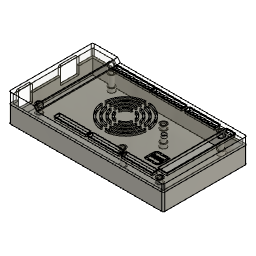
CaseArduino_MicaelMarques_2021.1 (Autodesk Fusion 360 design; units mm, degrees)
Autodesk Fusion 360 part; units mm, degrees
note: some values were not read from the file. Set by a fixed rule: which face or edge a step refers to.
sketch "Sketch1" plane through (0, 0, 0) normal (0, 0, 1) x (1, 0, 0)
  line L0 (-51.8, 28.67) -> (51.8, 28.67)
  line L1 (52.8, 27.67) -> (52.8, -27.67)
  line L2 (51.8, -28.67) -> (-51.8, -28.67)
  line L3 (-52.8, -27.67) -> (-52.8, 27.67)
  line L4 (-52.8, 28.67) -> (52.8, -28.67) construction
  line L5 (52.8, 28.67) -> (-52.8, -28.67) construction
  line L6 (-1.55, -22.32) -> (19.37, -22.32)
  line L7 (19.57, -22.52) -> (19.57, -25.53)
  line L8 (19.37, -25.73) -> (-1.55, -25.73)
  line L9 (-1.75, -25.53) -> (-1.75, -22.52)
  line L10 (21.31, -22.32) -> (42.23, -22.32)
  line L11 (42.43, -22.52) -> (42.43, -25.53)
  line L12 (42.23, -25.73) -> (21.31, -25.73)
  line L13 (21.11, -25.53) -> (21.11, -22.52)
  line L14 (-33.25, 25.94) -> (-7.85, 25.94)
  line L15 (-7.65, 25.74) -> (-7.65, 22.73)
  line L16 (-7.85, 22.53) -> (-33.25, 22.53)
  line L17 (-33.45, 22.73) -> (-33.45, 25.74)
  line L18 (-6.33, 25.94) -> (13.99, 25.94)
  line L19 (14.19, 25.74) -> (14.19, 22.73)
  line L20 (13.99, 22.53) -> (-6.33, 22.53)
  line L21 (-6.53, 22.73) -> (-6.53, 25.74)
  line L22 (16.53, 25.94) -> (36.85, 25.94)
  line L23 (37.05, 25.74) -> (37.05, 22.73)
  line L24 (36.85, 22.53) -> (16.53, 22.53)
  line L25 (16.33, 22.73) -> (16.33, 25.74)
  line L26 (41.69, 25.94) -> (47.24, 25.94)
  line L27 (47.44, 25.74) -> (47.44, -20.58)
  line L28 (47.24, -20.78) -> (41.69, -20.78)
  line L29 (41.49, -20.58) -> (41.49, 25.74)
  line L30 (-24.41, -22.32) -> (-3.49, -22.32)
  line L31 (-3.29, -22.52) -> (-3.29, -25.53)
  line L32 (-3.49, -25.73) -> (-24.41, -25.73)
  line L33 (-24.61, -25.53) -> (-24.61, -22.52)
  circle A0 centre (-36.81, -24.02) radius 2.2
  circle A1 centre (15.26, 9) radius 2.2
  circle A2 centre (15.26, -18.94) radius 2.2
  circle A3 centre (39.39, 24.24) radius 2.2
  circle A4 centre (45.74, -24.02) radius 2.2
  circle A5 centre (-36.81, -24.02) radius 1.5
  circle A6 centre (15.26, 9) radius 1.5
  circle A7 centre (15.26, -18.94) radius 1.5
  circle A8 centre (39.39, 24.24) radius 1.5
  circle A9 centre (45.74, -24.02) radius 1.5
  circle A10 centre (-35.54, 24.24) radius 2.2
  circle A11 centre (-35.54, 24.24) radius 1.5
  arc A12 (-33.25, 25.94) -> (-33.45, 25.74) centre (-33.25, 25.74) ccw
  arc A13 (-33.45, 22.73) -> (-33.25, 22.53) centre (-33.25, 22.73) ccw
  arc A14 (-7.85, 22.53) -> (-7.65, 22.73) centre (-7.85, 22.73) ccw
  arc A15 (-7.65, 25.74) -> (-7.85, 25.94) centre (-7.85, 25.74) ccw
  arc A16 (-6.33, 25.94) -> (-6.53, 25.74) centre (-6.33, 25.74) ccw
  arc A17 (-6.53, 22.73) -> (-6.33, 22.53) centre (-6.33, 22.73) ccw
  arc A18 (13.99, 22.53) -> (14.19, 22.73) centre (13.99, 22.73) ccw
  arc A19 (14.19, 25.74) -> (13.99, 25.94) centre (13.99, 25.74) ccw
  arc A20 (16.53, 25.94) -> (16.33, 25.74) centre (16.53, 25.74) ccw
  arc A21 (16.33, 22.73) -> (16.53, 22.53) centre (16.53, 22.73) ccw
  arc A22 (36.85, 22.53) -> (37.05, 22.73) centre (36.85, 22.73) ccw
  arc A23 (37.05, 25.74) -> (36.85, 25.94) centre (36.85, 25.74) ccw
  arc A24 (41.69, 25.94) -> (41.49, 25.74) centre (41.69, 25.74) ccw
  arc A25 (47.44, 25.74) -> (47.24, 25.94) centre (47.24, 25.74) ccw
  arc A26 (41.49, -20.58) -> (41.69, -20.78) centre (41.69, -20.58) ccw
  arc A27 (47.24, -20.78) -> (47.44, -20.58) centre (47.24, -20.58) ccw
  arc A28 (21.31, -22.32) -> (21.11, -22.52) centre (21.31, -22.52) ccw
  arc A29 (21.11, -25.53) -> (21.31, -25.73) centre (21.31, -25.53) ccw
  arc A30 (42.23, -25.73) -> (42.43, -25.53) centre (42.23, -25.53) ccw
  arc A31 (42.43, -22.52) -> (42.23, -22.32) centre (42.23, -22.52) ccw
  arc A32 (-1.55, -22.32) -> (-1.75, -22.52) centre (-1.55, -22.52) ccw
  arc A33 (-1.75, -25.53) -> (-1.55, -25.73) centre (-1.55, -25.53) ccw
  arc A34 (19.37, -25.73) -> (19.57, -25.53) centre (19.37, -25.53) ccw
  arc A35 (19.57, -22.52) -> (19.37, -22.32) centre (19.37, -22.52) ccw
  arc A36 (-24.41, -22.32) -> (-24.61, -22.52) centre (-24.41, -22.52) ccw
  arc A37 (-24.61, -25.53) -> (-24.41, -25.73) centre (-24.41, -25.53) ccw
  arc A38 (-3.49, -25.73) -> (-3.29, -25.53) centre (-3.49, -25.53) ccw
  arc A39 (-3.29, -22.52) -> (-3.49, -22.32) centre (-3.49, -22.52) ccw
  arc A40 (-33.75, 22.73) -> (-33.25, 22.23) centre (-33.25, 22.73) ccw
  line L34 (-7.85, 22.23) -> (-33.25, 22.23)
  arc A41 (-7.85, 22.23) -> (-7.35, 22.73) centre (-7.85, 22.73) ccw
  line L35 (-7.35, 25.74) -> (-7.35, 22.73)
  arc A42 (-7.35, 25.74) -> (-7.85, 26.24) centre (-7.85, 25.74) ccw
  line L36 (-33.25, 26.24) -> (-7.85, 26.24)
  arc A43 (-33.25, 26.24) -> (-33.75, 25.74) centre (-33.25, 25.74) ccw
  line L37 (-33.75, 22.73) -> (-33.75, 25.74)
  arc A44 (-6.83, 22.73) -> (-6.33, 22.23) centre (-6.33, 22.73) ccw
  line L38 (13.99, 22.23) -> (-6.33, 22.23)
  arc A45 (13.99, 22.23) -> (14.49, 22.73) centre (13.99, 22.73) ccw
  line L39 (14.49, 25.74) -> (14.49, 22.73)
  arc A46 (14.49, 25.74) -> (13.99, 26.24) centre (13.99, 25.74) ccw
  line L40 (-6.33, 26.24) -> (13.99, 26.24)
  arc A47 (-6.33, 26.24) -> (-6.83, 25.74) centre (-6.33, 25.74) ccw
  line L41 (-6.83, 22.73) -> (-6.83, 25.74)
  arc A48 (37.35, 25.74) -> (36.85, 26.24) centre (36.85, 25.74) ccw
  line L42 (16.53, 26.24) -> (36.85, 26.24)
  arc A49 (16.53, 26.24) -> (16.03, 25.74) centre (16.53, 25.74) ccw
  line L43 (16.03, 22.73) -> (16.03, 25.74)
  arc A50 (16.03, 22.73) -> (16.53, 22.23) centre (16.53, 22.73) ccw
  line L44 (36.85, 22.23) -> (16.53, 22.23)
  arc A51 (36.85, 22.23) -> (37.35, 22.73) centre (36.85, 22.73) ccw
  line L45 (37.35, 25.74) -> (37.35, 22.73)
  arc A52 (41.69, 26.24) -> (41.19, 25.74) centre (41.69, 25.74) ccw
  line L46 (41.19, -20.58) -> (41.19, 25.74)
  arc A53 (41.19, -20.58) -> (41.69, -21.08) centre (41.69, -20.58) ccw
  line L47 (47.24, -21.08) -> (41.69, -21.08)
  arc A54 (47.24, -21.08) -> (47.74, -20.58) centre (47.24, -20.58) ccw
  line L48 (47.74, 25.74) -> (47.74, -20.58)
  arc A55 (47.74, 25.74) -> (47.24, 26.24) centre (47.24, 25.74) ccw
  line L49 (41.69, 26.24) -> (47.24, 26.24)
  arc A56 (42.73, -22.52) -> (42.23, -22.02) centre (42.23, -22.52) ccw
  line L50 (21.31, -22.02) -> (42.23, -22.02)
  arc A57 (21.31, -22.02) -> (20.81, -22.52) centre (21.31, -22.52) ccw
  line L51 (20.81, -25.53) -> (20.81, -22.52)
  arc A58 (20.81, -25.53) -> (21.31, -26.03) centre (21.31, -25.53) ccw
  line L52 (42.23, -26.03) -> (21.31, -26.03)
  arc A59 (42.23, -26.03) -> (42.73, -25.53) centre (42.23, -25.53) ccw
  line L53 (42.73, -22.52) -> (42.73, -25.53)
  arc A60 (19.87, -22.52) -> (19.37, -22.02) centre (19.37, -22.52) ccw
  line L54 (-1.55, -22.02) -> (19.37, -22.02)
  arc A61 (-1.55, -22.02) -> (-2.05, -22.52) centre (-1.55, -22.52) ccw
  line L55 (-2.05, -25.53) -> (-2.05, -22.52)
  arc A62 (-2.05, -25.53) -> (-1.55, -26.03) centre (-1.55, -25.53) ccw
  line L56 (19.37, -26.03) -> (-1.55, -26.03)
  arc A63 (19.37, -26.03) -> (19.87, -25.53) centre (19.37, -25.53) ccw
  line L57 (19.87, -22.52) -> (19.87, -25.53)
  arc A64 (-2.99, -22.52) -> (-3.49, -22.02) centre (-3.49, -22.52) ccw
  line L58 (-24.41, -22.02) -> (-3.49, -22.02)
  arc A65 (-24.41, -22.02) -> (-24.91, -22.52) centre (-24.41, -22.52) ccw
  line L59 (-24.91, -25.53) -> (-24.91, -22.52)
  arc A66 (-24.91, -25.53) -> (-24.41, -26.03) centre (-24.41, -25.53) ccw
  line L60 (-3.49, -26.03) -> (-24.41, -26.03)
  arc A67 (-3.49, -26.03) -> (-2.99, -25.53) centre (-3.49, -25.53) ccw
  line L61 (-2.99, -22.52) -> (-2.99, -25.53)
  arc A68 (-51.8, 28.67) -> (-52.8, 27.67) centre (-51.8, 27.67) ccw
  arc A69 (-52.8, -27.67) -> (-51.8, -28.67) centre (-51.8, -27.67) ccw
  arc A70 (51.8, -28.67) -> (52.8, -27.67) centre (51.8, -27.67) ccw
  line L62 (51.3, -27.17) -> (-51.3, -27.17) construction
  line L63 (-51.3, -27.17) -> (-51.3, 27.17) construction
  line L64 (-51.3, 27.17) -> (51.3, 27.17) construction
  line L65 (51.3, 27.17) -> (51.3, -27.17) construction
  arc A71 (52.8, 27.67) -> (51.8, 28.67) centre (51.8, 27.67) ccw
  dimension "d1" = 105.6
  dimension "d2" = 57.34
  dimension "d3" = 2.94
  dimension "d6" = 3.41
  dimension "d9" = 10.37
  dimension "d10" = 21.32
  dimension "d11" = 1.54
  dimension "d12" = 21.32
  dimension "d15" = 1.54
  dimension "d16" = 21.32
  dimension "d17" = 5.36
  dimension "d18" = 5.95
  dimension "d19" = 7.89
  dimension "d20" = 46.72
  dimension "d21" = 4.44
  dimension "d22" = 20.72
  dimension "d23" = 2.14
  dimension "d24" = 20.72
  dimension "d25" = 1.12
  dimension "d26" = 25.8
  dimension "d27" = 3.41
  dimension "d28" = 2.73
  dimension "d30" = 4.4
  dimension "d31" = 4.4
  dimension "d32" = 4.4
  dimension "d33" = 4.4
  dimension "d34" = 4.4
  dimension "d36" = 3
  dimension "d37" = 3
  dimension "d38" = 3
  dimension "d39" = 3
  dimension "d40" = 3
  dimension "d41" = 13.41
  dimension "d42" = 4.43
  dimension "d43" = 7.06
  dimension "d44" = 4.65
  dimension "d45" = 9.73
  dimension "d46" = 37.54
  dimension "d47" = 37.54
  dimension "d48" = 19.67
  dimension "d49" = 4.65
  dimension "d50" = 15.99
  dimension "d51" = 12.2
  dimension "d53" = 4.4
  dimension "d54" = 3
  dimension "d55" = 4.43
  dimension "d56" = 17.26
  dimension "d57" = 1.5
  dimension "d131" = 0.2
  dimension "d132" = 0.2
  dimension "d133" = 0.2
  dimension "d134" = 0.2
  dimension "d135" = 0.2
  dimension "d136" = 0.2
  dimension "d137" = 0.2
  dimension "d138" = -0.3
  dimension "d139" = -0.3
  dimension "d140" = -0.3
  dimension "d141" = -0.3
  dimension "d142" = -0.3
  dimension "d143" = -0.3
  dimension "d144" = -0.3
  dimension "d158" = 1
  constraint horizontal L0
  constraint perpendicular L0 L1
  constraint parallel L0 L2
  constraint parallel L1 L3
  constraint coincident L4 origin
  constraint coincident L5 origin
  constraint horizontal L6
  constraint vertical L7
  constraint horizontal L8
  constraint vertical L9
  constraint horizontal L10
  constraint vertical L11
  constraint horizontal L12
  constraint vertical L13
  constraint horizontal L14
  constraint vertical L15
  constraint horizontal L16
  constraint vertical L17
  constraint horizontal L18
  constraint vertical L19
  constraint horizontal L20
  constraint vertical L21
  constraint horizontal L22
  constraint vertical L23
  constraint horizontal L24
  constraint vertical L25
  constraint horizontal L26
  constraint vertical L27
  constraint horizontal L28
  constraint vertical L29
  constraint collinear L8 L12
  constraint collinear L6 L10
  constraint horizontal L30
  constraint vertical L31
  constraint horizontal L32
  constraint vertical L33
  constraint collinear L8 L32
  constraint collinear L6 L30
  constraint collinear L18 L22
  constraint collinear L14 L22
  constraint collinear L20 L24
  constraint collinear L16 L24
  constraint concentric A0 A5
  constraint concentric A1 A6
  constraint concentric A2 A7
  constraint concentric A3 A8
  constraint concentric A4 A9
  constraint concentric A10 A11
  constraint tangent L14 A12
  constraint tangent L17 A12
  constraint tangent L16 A13
  constraint tangent L17 A13
  constraint equal A12 A13
  constraint tangent L16 A14
  constraint tangent L15 A14
  constraint equal A12 A14
  constraint tangent L14 A15
  constraint tangent L15 A15
  constraint equal A12 A15
  constraint tangent L18 A16
  constraint tangent L21 A16
  constraint tangent L20 A17
  constraint tangent L21 A17
  constraint equal A16 A17
  constraint tangent L19 A18
  constraint tangent L20 A18
  constraint equal A16 A18
  constraint tangent L18 A19
  constraint tangent L19 A19
  constraint equal A16 A19
  constraint tangent L22 A20
  constraint tangent L25 A20
  constraint tangent L24 A21
  constraint tangent L25 A21
  constraint equal A20 A21
  constraint tangent L23 A22
  constraint tangent L24 A22
  constraint equal A20 A22
  constraint tangent L22 A23
  constraint tangent L23 A23
  constraint equal A20 A23
  constraint tangent L26 A24
  constraint tangent L29 A24
  constraint tangent L26 A25
  constraint tangent L27 A25
  constraint equal A24 A25
  constraint tangent L28 A26
  constraint tangent L29 A26
  constraint equal A24 A26
  constraint tangent L27 A27
  constraint tangent L28 A27
  constraint equal A24 A27
  constraint tangent L10 A28
  constraint tangent L13 A28
  constraint tangent L12 A29
  constraint tangent L13 A29
  constraint equal A28 A29
  constraint tangent L11 A30
  constraint tangent L12 A30
  constraint equal A28 A30
  constraint tangent L10 A31
  constraint tangent L11 A31
  constraint equal A28 A31
  constraint tangent L6 A32
  constraint tangent L9 A32
  constraint tangent L8 A33
  constraint tangent L9 A33
  constraint equal A32 A33
  constraint tangent L7 A34
  constraint tangent L8 A34
  constraint equal A32 A34
  constraint tangent L6 A35
  constraint tangent L7 A35
  constraint equal A32 A35
  constraint tangent L30 A36
  constraint tangent L33 A36
  constraint tangent L32 A37
  constraint tangent L33 A37
  constraint equal A36 A37
  constraint tangent L31 A38
  constraint tangent L32 A38
  constraint equal A36 A38
  constraint tangent L30 A39
  constraint tangent L31 A39
  constraint equal A36 A39
  constraint coincident L4.start L0
  constraint tangent L0 A68
  constraint tangent L3 A68
  constraint coincident L5.end L3
  constraint tangent L3 A69
  constraint tangent L2 A69
  constraint equal A68 A69
  constraint coincident L4.end L2
  constraint coincident L4.end L1
  constraint tangent L2 A70
  constraint tangent L1 A70
  constraint equal A68 A70
  constraint coincident L5.start L0
  constraint coincident L5.start L1
  constraint tangent L0 A71
  constraint tangent L1 A71
  constraint equal A68 A71
  measures "d1" distance of L1 L3
  measures "d2" distance of L0 L2
  measures "d3" distance of L2 L12
  measures "d6" distance of L10 L12
  measures "d9" distance of L1 L11
  measures "d10" distance of L11 L13
  measures "d11" distance of L7 L13
  measures "d12" distance of L7 L9
  measures "d15" distance of L9 L31
  measures "d16" distance of L31 L33
  measures "d17" distance of L1 L27
  measures "d18" distance of L27 L29
  measures "d19" distance of L2 L28
  measures "d20" distance of L26 L28
  measures "d21" distance of L23 L29
  measures "d22" distance of L23 L25
  measures "d23" distance of L19 L25
  measures "d24" distance of L19 L21
  measures "d25" distance of L15 L21
  measures "d26" distance of L15 L17
  measures "d27" distance of L22 L24
  measures "d28" distance of L0 L22
  measures "d30" diameter of A0
  measures "d31" diameter of A1
  measures "d32" diameter of A2
  measures "d33" diameter of A3
  measures "d34" diameter of A4
  measures "d36" diameter of A5
  measures "d37" diameter of A6
  measures "d38" diameter of A7
  measures "d39" diameter of A8
  measures "d40" diameter of A9
  measures "d41" distance of L1 A3.centre
  measures "d42" distance of L0 A3.centre
  measures "d43" distance of L1 A4.centre
  measures "d44" distance of L2 A4.centre
  measures "d45" distance of L2 A2.centre
  measures "d46" distance of L1 A2.centre
  measures "d47" distance of L1 A1.centre
  measures "d48" distance of L0 A1.centre
  measures "d49" distance of L2 A0.centre
  measures "d50" distance of L3 A0.centre
  measures "d51" distance of L33 A0.centre
  measures "d53" diameter of A10
  measures "d54" diameter of A11
  measures "d55" distance of L0 A10.centre
  measures "d56" distance of L3 A10.centre
  measures "d131" radius of A12
  measures "d132" radius of A16
  measures "d133" radius of A20
  measures "d134" radius of A24
  measures "d135" radius of A28
  measures "d136" radius of A32
  measures "d137" radius of A36
  measures "d158" radius of A68
extrude "Extrude1" add sketch "Sketch1" along normal blind 19 contours L0 L1 L2 L3 A68 A69 A70 A71 | L6 L7 L8 L9 A32 A33 A34 A35 | L10 L11 L12 L13 A28 A29 A30 A31 | L14 L15 L16 L17 A10 A12 A13 A14 A15 A40 L34 A41 L35 A42 L36 A43 L37 | L14 L15 L16 L17 A10 A12 A13 A14 A15 | L17 A10 | L17 A10 L37 | A10 L37 | L18 L19 L20 L21 A16 A17 A18 A19 | L22 L23 L24 L25 A20 A21 A22 A23 | L26 L27 L28 L29 A3 A24 A25 A26 A27 A52 L46 A53 L47 A54 L48 A55 L49 | L26 L27 L28 L29 A3 A24 A25 A26 A27 | L29 A3 | L29 A3 L46 | A3 L45 L46 | A3 L45 | A3 A48 L42 A49 L43 A50 L44 A51 L45 | L30 L31 L32 L33 A36 A37 A38 A39 | A0 | A1 | A2 | A4 | A5 | A6 | A7 | A8 | A9 | A11 | A44 L38 A45 L39 A46 L40 A47 L41 | A56 L50 A57 L51 A58 L52 A59 L53 | A60 L54 A61 L55 A62 L56 A63 L57 | A64 L58 A65 L59 A66 L60 A67 L61 makes body 1
sketch "Sketch2" plane through (0, -28.67, 0) normal (0, -1, 0) x (1, 0, 0)
  line L0 (-51.8, 0) -> (51.8, 0)
  line L1 (51.8, 19) -> (-51.8, 19)
  line L2 (61, 16.5) -> (-33.95, 16.5)
  line L3 (-36.45, 38.5) -> (59, 38.5)
  line L4 (61, 16.5) -> (61, 38)
  line L5 (61, 38.5) -> (59, 38.5)
  line L6 (61, 38) -> (61, 38.5)
  line L7 (-33.95, 16.5) -> (-36.45, 20.0211)
  line L8 (-36.45, 20.0211) -> (-36.45, 38.5)
  line L9 (51.8, 0) -> (51.8, 19)
  line L10 (-51.8, 19) -> (-51.8, 0)
  dimension "d60" = 16.5
  dimension "d63" = 2.5
  constraint perpendicular L2 L4
  constraint perpendicular L4 L5
  constraint perpendicular L5 L6
  measures "d60" distance of L0 L2
  measures "d63" horizontal distance of L2.end L7.end
extrude "Extrude2" cut sketch "Sketch2" against normal blind 80 contours L1 L2 L3 L4 L5 L6 L7 L8 L9 | L1 L2 L7 L9 bodies 1
shell "Shell1" thickness 1.5 removed faces 0 bodies 1
ref_plane "WorkPlane1" through (0, 0, 11.5) normal (0, 0, -1) x (-1, 0, 0)
split "Split1" by plane through (0, 0, 11.5) normal (0, 0, -1) bodies 1 makes body 2 at (17.2667, -9.5567, 0)
extrude "Extrude3" add sketch "Sketch1" along normal blind 13 from surface at 1.5 contours A5 | A6 | A7 | A8 | A9 | A11 bodies 2
extrude "Extrude4" add sketch "Sketch1" along normal blind 2.7 from surface at 1.5 contours L17 A10 | L17 A10 L37 | A10 L37 | L29 A3 | L29 A3 L46 | A3 L45 L46 | A3 L45 | A0 | A1 | A2 | A4 bodies 2
chamfer "Chamfer1" distance 0.5 angle 45 6 edges at (-38.2085, -24.5624, 14.5) (-36.9385, 23.6976, 14.5) (13.8615, 8.4576, 14.5) (13.8615, -19.4824, 14.5) (37.9915, 23.6976, 14.5) (44.3415, -24.5624, 14.5) on bodies 2
extrude "Extrude5" add sketch "Sketch1" against normal blind 3 from surface at 15 contours L29 A3 L46 | A3 L45 L46 | A3 L45 | A1 | A2 | A4 bodies 1
extrude "Extrude6" add sketch "Sketch1" against normal blind 5.5 from surface at 17.5 contours L17 A10 | L17 A10 L37 | A10 L37 | A0 bodies 1
extrude "Extrude7" cut sketch "Sketch2" against normal blind 117 contours L1 L2 L3 L4 L5 L6 L7 L8 L9 | L1 L2 L7 L9 bodies 1
extrude "Extrude8" cut sketch "Sketch1" along normal blind 34 contours L6 L7 L8 L9 A32 A33 A34 A35 | L10 L11 L12 L13 A28 A29 A30 A31 | L14 L15 L16 L17 A10 A12 A13 A14 A15 | L17 A10 | L18 L19 L20 L21 A16 A17 A18 A19 | L22 L23 L24 L25 A20 A21 A22 A23 | L26 L27 L28 L29 A3 A24 A25 A26 A27 | L29 A3 | L30 L31 L32 L33 A36 A37 A38 A39 bodies 1
sketch "Sketch3" plane through (0, 0, 16.5) normal (0, 0, 1) x (-1, 0, 0)
  line L0 (-16.33, -22.73) -> (-16.33, -25.74)
  line L1 (-16.53, -25.94) -> (-36.85, -25.94)
  line L2 (-37.05, -25.74) -> (-37.05, -22.73)
  line L3 (-36.85, -22.53) -> (-16.53, -22.53)
  line L4 (24.61, 25.53) -> (24.61, 22.52)
  line L5 (24.41, 22.32) -> (3.49, 22.32)
  line L6 (3.29, 22.52) -> (3.29, 25.53)
  line L7 (3.49, 25.73) -> (24.41, 25.73)
  line L8 (-41.49, 20.58) -> (-41.49, -25.74)
  line L9 (-41.69, -25.94) -> (-47.24, -25.94)
  line L10 (-47.44, -25.74) -> (-47.44, 20.58)
  line L11 (-47.24, 20.78) -> (-41.69, 20.78)
  line L12 (6.53, -22.73) -> (6.53, -25.74)
  line L13 (6.33, -25.94) -> (-13.99, -25.94)
  line L14 (-14.19, -25.74) -> (-14.19, -22.73)
  line L15 (-13.99, -22.53) -> (6.33, -22.53)
  line L16 (1.75, 25.53) -> (1.75, 22.52)
  line L17 (1.55, 22.32) -> (-19.37, 22.32)
  line L18 (-19.57, 22.52) -> (-19.57, 25.53)
  line L19 (-19.37, 25.73) -> (1.55, 25.73)
  line L20 (-21.11, 25.53) -> (-21.11, 22.52)
  line L21 (-21.31, 22.32) -> (-42.23, 22.32)
  line L22 (-42.43, 22.52) -> (-42.43, 25.53)
  line L23 (-42.23, 25.73) -> (-21.31, 25.73)
  line L24 (33.45, -22.73) -> (33.45, -25.74)
  line L25 (33.25, -25.94) -> (7.85, -25.94)
  line L26 (7.65, -25.74) -> (7.65, -22.73)
  line L27 (7.85, -22.53) -> (33.25, -22.53)
  line L28 (33.95, -28.67) -> (33.95, 28.67)
  line L29 (33.95, 28.67) -> (-51.8, 28.67)
  line L30 (-52.8, 27.67) -> (-52.8, -27.67)
  line L31 (-51.8, -28.67) -> (33.95, -28.67)
  line L32 (1.23, -45) -> (1.23, 40) construction
  line L33 (70, 0.5) -> (-65, 0.5) construction
  line L34 (52.8, -30.2) -> (52.8, 50) construction
  line L35 (53, 28.67) -> (-69, 28.67) construction
  circle A0 centre (1.23, 0.5) radius 15 construction
  circle A1 centre (1.23, 0.5) radius 12 construction
  circle A2 centre (1.23, 0.5) radius 9 construction
  circle A3 centre (1.23, 0.5) radius 6 construction
  line L36 (2.73, -38) -> (2.73, 36) construction
  line L37 (-0.27, -37) -> (-0.27, 40) construction
  line L38 (70, 2) -> (-14.1923, 2) construction
  line L39 (70, -1) -> (-15, -1) construction
  arc A4 (-14.1923, -1.05) -> (-0.32, -14.9223) centre (1.23, 0.5) ccw
  arc A5 (-13.1973, -0.95) -> (-14.1923, -1.05) centre (-13.6948, -1) ccw
  arc A6 (-13.1973, -0.95) -> (-0.22, -13.9273) centre (1.23, 0.5) ccw
  arc A7 (-0.32, -14.9223) -> (-0.22, -13.9273) centre (-0.27, -14.4248) ccw
  arc A8 (-13.6948, -1) -> (-0.27, -14.4248) centre (1.23, 0.5) ccw construction
  arc A9 (-11.172, -1.0625) -> (-0.3325, -11.902) centre (1.23, 0.5) ccw
  arc A10 (-10.1798, -0.9375) -> (-11.172, -1.0625) centre (-10.6759, -1) ccw
  arc A11 (-10.1798, -0.9375) -> (-0.2075, -10.9098) centre (1.23, 0.5) ccw
  arc A12 (-0.3325, -11.902) -> (-0.2075, -10.9098) centre (-0.27, -11.4059) ccw
  arc A13 (-10.6759, -1) -> (-0.27, -11.4059) centre (1.23, 0.5) ccw construction
  arc A14 (-8.1371, -1.0833) -> (-0.3533, -8.8671) centre (1.23, 0.5) ccw
  arc A15 (-7.1511, -0.9167) -> (-8.1371, -1.0833) centre (-7.6441, -1) ccw
  arc A16 (-7.1511, -0.9167) -> (-0.1867, -7.8811) centre (1.23, 0.5) ccw
  arc A17 (-0.3533, -8.8671) -> (-0.1867, -7.8811) centre (-0.27, -8.3741) ccw
  arc A18 (-7.6441, -1) -> (-0.27, -8.3741) centre (1.23, 0.5) ccw construction
  arc A19 (-5.0636, -1.125) -> (-0.395, -5.7936) centre (1.23, 0.5) ccw
  arc A20 (-4.0954, -0.875) -> (-5.0636, -1.125) centre (-4.5795, -1) ccw
  arc A21 (-4.0954, -0.875) -> (-0.145, -4.8254) centre (1.23, 0.5) ccw
  arc A22 (-0.395, -5.7936) -> (-0.145, -4.8254) centre (-0.27, -5.3095) ccw
  arc A23 (-4.5795, -1) -> (-0.27, -5.3095) centre (1.23, 0.5) ccw construction
  arc A24 (2.6467, -7.8811) -> (9.6111, -0.9167) centre (1.23, 0.5) ccw
  arc A25 (2.73, -8.3741) -> (10.1041, -1) centre (1.23, 0.5) ccw construction
  arc A26 (2.73, -11.4059) -> (13.1359, -1) centre (1.23, 0.5) ccw construction
  arc A27 (2.8133, -8.8671) -> (10.5971, -1.0833) centre (1.23, 0.5) ccw
  arc A28 (2.6675, -10.9098) -> (2.7925, -11.902) centre (2.73, -11.4059) ccw
  arc A29 (2.68, -13.9273) -> (2.78, -14.9223) centre (2.73, -14.4248) ccw
  arc A30 (2.605, -4.8254) -> (2.855, -5.7936) centre (2.73, -5.3095) ccw
  arc A31 (2.6467, -7.8811) -> (2.8133, -8.8671) centre (2.73, -8.3741) ccw
  arc A32 (7.5236, -1.125) -> (6.5554, -0.875) centre (7.0395, -1) ccw
  arc A33 (2.73, -5.3095) -> (7.0395, -1) centre (1.23, 0.5) ccw construction
  arc A34 (16.6523, -1.05) -> (15.6573, -0.95) centre (16.1548, -1) ccw
  arc A35 (10.5971, -1.0833) -> (9.6111, -0.9167) centre (10.1041, -1) ccw
  arc A36 (13.632, -1.0625) -> (12.6398, -0.9375) centre (13.1359, -1) ccw
  arc A37 (2.605, -4.8254) -> (6.5554, -0.875) centre (1.23, 0.5) ccw
  arc A38 (2.78, -14.9223) -> (16.6523, -1.05) centre (1.23, 0.5) ccw
  arc A39 (2.73, -14.4248) -> (16.1548, -1) centre (1.23, 0.5) ccw construction
  arc A40 (2.6675, -10.9098) -> (12.6398, -0.9375) centre (1.23, 0.5) ccw
  arc A41 (2.68, -13.9273) -> (15.6573, -0.95) centre (1.23, 0.5) ccw
  arc A42 (2.855, -5.7936) -> (7.5236, -1.125) centre (1.23, 0.5) ccw
  arc A43 (2.7925, -11.902) -> (13.632, -1.0625) centre (1.23, 0.5) ccw
  arc A44 (9.6111, 1.9167) -> (2.6467, 8.8811) centre (1.23, 0.5) ccw
  arc A45 (10.1041, 2) -> (2.73, 9.3741) centre (1.23, 0.5) ccw construction
  arc A46 (13.1359, 2) -> (2.73, 12.4059) centre (1.23, 0.5) ccw construction
  arc A47 (10.5971, 2.0833) -> (2.8133, 9.8671) centre (1.23, 0.5) ccw
  arc A48 (12.6398, 1.9375) -> (13.632, 2.0625) centre (13.1359, 2) ccw
  arc A49 (15.6573, 1.95) -> (16.6523, 2.05) centre (16.1548, 2) ccw
  arc A50 (6.5554, 1.875) -> (7.5236, 2.125) centre (7.0395, 2) ccw
  arc A51 (9.6111, 1.9167) -> (10.5971, 2.0833) centre (10.1041, 2) ccw
  arc A52 (2.855, 6.7936) -> (2.605, 5.8254) centre (2.73, 6.3095) ccw
  arc A53 (7.0395, 2) -> (2.73, 6.3095) centre (1.23, 0.5) ccw construction
  arc A54 (2.78, 15.9223) -> (2.68, 14.9273) centre (2.73, 15.4248) ccw
  arc A55 (2.8133, 9.8671) -> (2.6467, 8.8811) centre (2.73, 9.3741) ccw
  arc A56 (2.7925, 12.902) -> (2.6675, 11.9098) centre (2.73, 12.4059) ccw
  arc A57 (6.5554, 1.875) -> (2.605, 5.8254) centre (1.23, 0.5) ccw
  arc A58 (16.6523, 2.05) -> (2.78, 15.9223) centre (1.23, 0.5) ccw
  arc A59 (16.1548, 2) -> (2.73, 15.4248) centre (1.23, 0.5) ccw construction
  arc A60 (12.6398, 1.9375) -> (2.6675, 11.9098) centre (1.23, 0.5) ccw
  arc A61 (15.6573, 1.95) -> (2.68, 14.9273) centre (1.23, 0.5) ccw
  arc A62 (7.5236, 2.125) -> (2.855, 6.7936) centre (1.23, 0.5) ccw
  arc A63 (13.632, 2.0625) -> (2.7925, 12.902) centre (1.23, 0.5) ccw
  arc A64 (-0.1867, 8.8811) -> (-7.1511, 1.9167) centre (1.23, 0.5) ccw
  arc A65 (-0.27, 9.3741) -> (-7.6441, 2) centre (1.23, 0.5) ccw construction
  arc A66 (-0.27, 12.4059) -> (-10.6759, 2) centre (1.23, 0.5) ccw construction
  arc A67 (-0.3533, 9.8671) -> (-8.1371, 2.0833) centre (1.23, 0.5) ccw
  arc A68 (-0.2075, 11.9098) -> (-0.3325, 12.902) centre (-0.27, 12.4059) ccw
  arc A69 (-0.22, 14.9273) -> (-0.32, 15.9223) centre (-0.27, 15.4248) ccw
  arc A70 (-0.145, 5.8254) -> (-0.395, 6.7936) centre (-0.27, 6.3095) ccw
  arc A71 (-0.1867, 8.8811) -> (-0.3533, 9.8671) centre (-0.27, 9.3741) ccw
  arc A72 (-5.0636, 2.125) -> (-4.0954, 1.875) centre (-4.5795, 2) ccw
  arc A73 (-0.27, 6.3095) -> (-4.5795, 2) centre (1.23, 0.5) ccw construction
  arc A74 (-14.1923, 2.05) -> (-13.1973, 1.95) centre (-13.6948, 2) ccw
  arc A75 (-8.1371, 2.0833) -> (-7.1511, 1.9167) centre (-7.6441, 2) ccw
  arc A76 (-11.172, 2.0625) -> (-10.1798, 1.9375) centre (-10.6759, 2) ccw
  arc A77 (-0.145, 5.8254) -> (-4.0954, 1.875) centre (1.23, 0.5) ccw
  arc A78 (-0.32, 15.9223) -> (-14.1923, 2.05) centre (1.23, 0.5) ccw
  arc A79 (-0.27, 15.4248) -> (-13.6948, 2) centre (1.23, 0.5) ccw construction
  arc A80 (-0.2075, 11.9098) -> (-10.1798, 1.9375) centre (1.23, 0.5) ccw
  arc A81 (-0.22, 14.9273) -> (-13.1973, 1.95) centre (1.23, 0.5) ccw
  arc A82 (-0.395, 6.7936) -> (-5.0636, 2.125) centre (1.23, 0.5) ccw
  arc A83 (-0.3325, 12.902) -> (-11.172, 2.0625) centre (1.23, 0.5) ccw
  circle A84 centre (-23.38, -1.35) radius 1.5
  line L40 (-39.727, 10.753) -> (-39.727, 17.247)
  line L41 (-37.727, 19.247) -> (-30.273, 19.247)
  line L42 (-30.273, 10.753) -> (-39.727, 19.247) construction
  line L43 (-39.727, 10.753) -> (-30.273, 19.247) construction
  arc A85 (-32.273, 10.753) -> (-30.273, 12.753) centre (-32.273, 12.753) ccw
  arc A86 (-37.727, 19.247) -> (-39.727, 17.247) centre (-37.727, 17.247) ccw
  arc A87 (-37.727, 18.247) -> (-38.727, 17.247) centre (-37.727, 17.247) ccw
  line L44 (-38.727, 11.753) -> (-38.727, 17.247)
  arc A88 (-32.273, 11.753) -> (-31.273, 12.753) centre (-32.273, 12.753) ccw
  line L45 (-31.273, 17.747) -> (-31.273, 12.753)
  line L46 (-37.727, 18.247) -> (-31.273, 18.247)
  line L47 (-38.727, 11.753) -> (-38.727, 10.753)
  line L48 (-38.227, 11.753) -> (-38.227, 10.753)
  line L49 (-31.273, 18.247) -> (-30.273, 18.247)
  line L50 (-31.273, 17.747) -> (-30.273, 17.747)
  line L51 (-30.273, 19.247) -> (-30.273, 18.247)
  line L52 (-30.273, 17.747) -> (-30.273, 12.753)
  line L53 (-32.273, 11.753) -> (-38.227, 11.753)
  line L54 (-38.614, 11.753) -> (-38.727, 11.753)
  line L55 (-32.273, 10.753) -> (-38.227, 10.753)
  line L56 (-38.727, 10.753) -> (-39.727, 10.753)
  line L57 (-32.4719, 16.6174) -> (-37.5801, 16.6174) construction
  line L58 (-37.5801, 16.6174) -> (-37.5801, 13.6444) construction
  line L59 (-37.5801, 13.6444) -> (-32.4719, 13.6444) construction
  line L60 (-32.4719, 13.6444) -> (-32.4719, 16.6174) construction
  arc A89 (-16.33, -22.73) -> (-16.53, -22.53) centre (-16.53, -22.73) ccw
  arc A90 (-16.53, -25.94) -> (-16.33, -25.74) centre (-16.53, -25.74) ccw
  arc A91 (-37.05, -25.74) -> (-36.85, -25.94) centre (-36.85, -25.74) ccw
  arc A92 (-36.85, -22.53) -> (-37.05, -22.73) centre (-36.85, -22.73) ccw
  arc A93 (24.61, 25.53) -> (24.41, 25.73) centre (24.41, 25.53) ccw
  arc A94 (24.41, 22.32) -> (24.61, 22.52) centre (24.41, 22.52) ccw
  arc A95 (3.29, 22.52) -> (3.49, 22.32) centre (3.49, 22.52) ccw
  arc A96 (3.49, 25.73) -> (3.29, 25.53) centre (3.49, 25.53) ccw
  arc A97 (-41.69, -25.94) -> (-41.49, -25.74) centre (-41.69, -25.74) ccw
  arc A98 (-47.44, -25.74) -> (-47.24, -25.94) centre (-47.24, -25.74) ccw
  arc A99 (-47.24, 20.78) -> (-47.44, 20.58) centre (-47.24, 20.58) ccw
  arc A100 (-41.49, 20.58) -> (-41.69, 20.78) centre (-41.69, 20.58) ccw
  arc A101 (6.53, -22.73) -> (6.33, -22.53) centre (6.33, -22.73) ccw
  arc A102 (6.33, -25.94) -> (6.53, -25.74) centre (6.33, -25.74) ccw
  arc A103 (-14.19, -25.74) -> (-13.99, -25.94) centre (-13.99, -25.74) ccw
  arc A104 (-13.99, -22.53) -> (-14.19, -22.73) centre (-13.99, -22.73) ccw
  arc A105 (1.75, 25.53) -> (1.55, 25.73) centre (1.55, 25.53) ccw
  arc A106 (1.55, 22.32) -> (1.75, 22.52) centre (1.55, 22.52) ccw
  arc A107 (-19.57, 22.52) -> (-19.37, 22.32) centre (-19.37, 22.52) ccw
  arc A108 (-19.37, 25.73) -> (-19.57, 25.53) centre (-19.37, 25.53) ccw
  arc A109 (-21.11, 25.53) -> (-21.31, 25.73) centre (-21.31, 25.53) ccw
  arc A110 (-21.31, 22.32) -> (-21.11, 22.52) centre (-21.31, 22.52) ccw
  arc A111 (-42.43, 22.52) -> (-42.23, 22.32) centre (-42.23, 22.52) ccw
  arc A112 (-42.23, 25.73) -> (-42.43, 25.53) centre (-42.23, 25.53) ccw
  arc A113 (33.45, -22.73) -> (33.25, -22.53) centre (33.25, -22.73) ccw
  arc A114 (33.25, -25.94) -> (33.45, -25.74) centre (33.25, -25.74) ccw
  arc A115 (7.65, -25.74) -> (7.85, -25.94) centre (7.85, -25.74) ccw
  arc A116 (7.85, -22.53) -> (7.65, -22.73) centre (7.85, -22.73) ccw
  arc A117 (-51.8, 28.67) -> (-52.8, 27.67) centre (-51.8, 27.67) ccw
  arc A118 (-52.8, -27.67) -> (-51.8, -28.67) centre (-51.8, -27.67) ccw
  point P0 (-35, 15)
  dimension "d88" = 51.57
  dimension "d90" = 28.17
  dimension "d91" = 30
  dimension "d92" = 24
  dimension "d93" = 18
  dimension "d94" = 12
  dimension "d95" = 1.5
  dimension "d96" = 1.5
  dimension "d97" = 1.5
  dimension "d98" = 1.5
  dimension "d100" = 360
  dimension "d101" = 3
  dimension "d102" = 29.42
  dimension "d103" = 30.02
  dimension "d104" = 2
  dimension "d105" = 2
  dimension "d107" = 0.5
  dimension "d108" = 0.5
  dimension "d110" = 2.5
  text T0 "MM" font "Arial Black" height 2.5 bold align centre top in box 5.1082 x 2.973 at (-32.4719, 16.6174) x (-1, 0) y (0, -1) spacing 1 kerned
  constraint vertical L32
  constraint perpendicular L30 L33
  constraint perpendicular L33 L34
  constraint perpendicular L34 L35
  constraint coincident L33 A0.centre
  constraint coincident L32 A0.centre
  constraint concentric A0 A1
  constraint concentric A0 A2
  constraint concentric A2 A3
  constraint perpendicular L7 L36
  constraint parallel L32 L37
  constraint perpendicular L30 L38
  constraint perpendicular L30 L39
  constraint tangent A4 A5
  constraint tangent A5 A6
  constraint tangent A6 A7
  constraint tangent A4 A7
  constraint coincident A0.centre A1.centre
  constraint coincident L39 A5.centre
  constraint coincident A0 A7.centre
  constraint coincident L37 A7.centre
  constraint tangent A9 A10
  constraint tangent A10 A11
  constraint tangent A11 A12
  constraint tangent A9 A12
  constraint coincident L39 A10.centre
  constraint coincident L37 A12.centre
  constraint coincident A1 A12.centre
  constraint tangent A14 A15
  constraint tangent A15 A16
  constraint tangent A16 A17
  constraint tangent A14 A17
  constraint coincident L39 A15.centre
  constraint coincident A2 A17.centre
  constraint coincident L37 A17.centre
  constraint tangent A19 A20
  constraint tangent A20 A21
  constraint tangent A21 A22
  constraint tangent A19 A22
  constraint coincident L39 A20.centre
  constraint coincident A3 A20.centre
  constraint coincident L37 A22.centre
  constraint horizontal L55
  constraint perpendicular L40 L55
  constraint parallel L41 L55
  constraint parallel L40 L51
  constraint coincident L42 P0
  constraint coincident L43 P0
  constraint coincident L42.start L55
  constraint coincident L42.start L51
  constraint tangent A85 L55
  constraint tangent A85 L51
  constraint coincident L42.end L41
  constraint coincident L42.end L40
  constraint tangent L41 A86
  constraint tangent L40 A86
  constraint perpendicular L47 L53
  constraint perpendicular L48 L55
  constraint perpendicular L45 L49
  constraint perpendicular L45 L50
  constraint coincident L50.end L51
  constraint collinear L51 L52
  constraint concentric A86 A87
  constraint parallel L40 L44
  constraint parallel L53 L55
  constraint concentric A85 A88
  constraint parallel L41 L46
  constraint tangent A88 L45
  constraint tangent A87 L46
  constraint tangent A87 L44
  constraint tangent A88 L53
  constraint coincident L43 L54.start
  constraint collinear L53 L54
  constraint collinear L55 L56
  measures "d88" distance of L32 L34
  measures "d90" distance of L33 L35
  measures "d91" diameter of A0
  measures "d92" diameter of A1
  measures "d93" diameter of A2
  measures "d94" diameter of A3
  measures "d95" distance of L32 L36
  measures "d96" distance of L32 L37
  measures "d97" distance of L33 L39
  measures "d98" distance of L33 L38
  measures "d101" diameter of A84
  measures "d102" distance of L30 A84.centre
  measures "d103" distance of L35 A84.centre
  measures "d104" radius of A85
  measures "d105" radius of A86
  measures "d107" distance of L47 L48
  measures "d108" distance of L46.end L50
extrude "Extrude9" cut sketch "Sketch3" against normal blind 10 contours A4 A5 A6 A7 | A9 A10 A11 A12 | A14 A15 A16 A17 | A19 A20 A21 A22 | A24 A27 A31 A35 | A28 A36 A40 A43 | A29 A34 A38 A41 | A30 A32 A37 A42 | A44 A47 A51 A55 | A48 A56 A60 A63 | A49 A54 A58 A61 | A50 A52 A57 A62 | A64 A67 A71 A75 | A68 A76 A80 A83 | A69 A74 A78 A81 | A70 A72 A77 A82 | A84 bodies 1
extrude "Extrude10" cut sketch "Sketch3" sketch "Sketch3" against normal blind 0.2 contours L40 L41 A86 A87 L44 L46 L47 L49 L51 L56 | A85 A88 L45 L48 L50 L52 L53 L55 of sketch 2 text T0 bodies 1
ref_plane "WorkPlane3" through (-55.8, 0, 9.5) normal (-1, 0, 0) x (0, -1, 0)
sketch "Sketch4" plane through (-55.8, 0, 5.75) normal (-1, 0, 0) x (0, 1, 0)
  line L0 (16.98, -11.61) -> (5.94, -11.61)
  line L1 (5.14, -10.81) -> (5.14, -0.39)
  line L2 (5.14, -0.39) -> (17.78, -0.39)
  line L3 (17.78, -0.39) -> (17.78, -10.81)
  line L4 (-14.89, -11.56) -> (-22.89, -11.56)
  line L5 (-23.69, -10.76) -> (-23.69, 0.04)
  line L6 (-23.69, 0.04) -> (-14.09, 0.04)
  line L7 (-14.09, 0.04) -> (-14.09, -10.76)
  line L8 (29.5, 5.75) -> (-36, 5.75) construction
  line L9 (28.67, -13.3) -> (28.67, 12.2963) construction
  arc A0 (16.98, -11.61) -> (17.78, -10.81) centre (16.98, -10.81) ccw
  arc A1 (5.14, -10.81) -> (5.94, -11.61) centre (5.94, -10.81) ccw
  line L10 (-28.67, -13.31) -> (-28.67, 12.7156) construction
  arc A2 (-14.89, -11.56) -> (-14.09, -10.76) centre (-14.89, -10.76) ccw
  arc A3 (-23.69, -10.76) -> (-22.89, -11.56) centre (-22.89, -10.76) ccw
  dimension "d117" = 6.14
  dimension "d118" = 11.22
  dimension "d119" = 0.8
  dimension "d120" = 0.8
  dimension "d121" = 12.64
  dimension "d122" = 10.89
  dimension "d123" = 9.6
  dimension "d124" = 5.71
  dimension "d125" = 11.6
  dimension "d126" = 4.98
  dimension "d127" = 0.8
  dimension "d128" = 0.8
  constraint horizontal L0
  constraint vertical L1
  constraint horizontal L2
  constraint vertical L3
  constraint horizontal L4
  constraint vertical L5
  constraint horizontal L6
  constraint vertical L7
  constraint horizontal L8
  constraint perpendicular L8 L9
  constraint tangent L0 A0
  constraint tangent L3 A0
  constraint tangent L0 A1
  constraint tangent L1 A1
  constraint perpendicular L8 L10
  constraint tangent L4 A2
  constraint tangent L7 A2
  constraint tangent L4 A3
  constraint tangent L5 A3
  measures "d117" distance of L2 L8
  measures "d118" distance of L0 L2
  measures "d119" radius of A0
  measures "d120" radius of A1
  measures "d121" distance of L1 L3
  measures "d122" distance of L3 L9
  measures "d123" distance of L5 L7
  measures "d124" distance of L6 L8
  measures "d125" distance of L4 L6
  measures "d126" distance of L5 L10
  measures "d127" radius of A2
  measures "d128" radius of A3
extrude "Extrude11" cut sketch "Sketch4" against normal blind 10 bodies 1 2
extrude "Extrude12" add sketch "Sketch1" along normal blind 0.3 from surface at 16.5 contours L14 L15 L16 L17 A10 A12 A13 A14 A15 A40 L34 A41 L35 A42 L36 A43 L37 | L17 A10 L37 | L26 L27 L28 L29 A3 A24 A25 A26 A27 A52 L46 A53 L47 A54 L48 A55 L49 | L29 A3 L46 | A3 A48 L42 A49 L43 A50 L44 A51 L45 | A44 L38 A45 L39 A46 L40 A47 L41 | A56 L50 A57 L51 A58 L52 A59 L53 | A60 L54 A61 L55 A62 L56 A63 L57 | A64 L58 A65 L59 A66 L60 A67 L61 bodies 1
sketch "Sketch5" plane through (0, 0, 0) normal (0, 0, 1) x (1, 0, 0)
  line L0 (-70, -18.67) -> (65, -18.67) construction
  line L1 (42.8, -40) -> (42.8, 36.7218) construction
  line L2 (60, 18.67) -> (-60, 18.67) construction
  line L3 (-42.8, -35) -> (-42.8, 35) construction
  line L4 (-52.8, -27.67) -> (-52.8, 27.67)
  line L5 (52.8, 27.67) -> (52.8, -27.67)
  line L6 (51.8, -28.67) -> (-51.8, -28.67)
  line L7 (-51.8, 28.67) -> (51.8, 28.67)
  circle A0 centre (-42.8, -18.67) radius 4.5
  circle A1 centre (42.8, -18.67) radius 4.5
  circle A2 centre (-42.8, 18.67) radius 4.5
  circle A3 centre (42.8, 18.67) radius 4.5
  dimension "d148" = 10
  dimension "d149" = 10
  dimension "d150" = 10
  dimension "d151" = 10
  dimension "d152" = 9
  dimension "d153" = 9
  dimension "d154" = 9
  dimension "d155" = 9
  constraint horizontal L0
  constraint vertical L1
  constraint perpendicular L1 L2
  constraint perpendicular L2 L3
  constraint coincident L0 A0.centre
  constraint coincident L3 A0.centre
  constraint coincident L0 A1.centre
  constraint coincident L1 A1.centre
  constraint coincident L2 A2.centre
  constraint coincident L3 A2.centre
  constraint coincident L2 A3.centre
  constraint coincident L1 A3.centre
  measures "d148" distance of L3 L4
  measures "d149" distance of L1 L5
  measures "d150" distance of L0 L6
  measures "d151" distance of L2 L7
  measures "d152" diameter of A0
  measures "d153" diameter of A1
  measures "d154" diameter of A2
  measures "d155" diameter of A3
extrude "Extrude13" add sketch "Sketch5" against normal blind 0.5 bodies 2
move_body "Move1" bodies 2 to x (1, 0, 0) y (0, 1, 0) z (0, 0, 1) at (1, 0, 0)
move_body "Move2" bodies 2 to x (1, 0, 0) y (0, 1, 0) z (0, 0, 1) at (-0.5, 0, 0)
move_body "Move3" bodies 1 to x (1, 0, 0) y (0, 1, 0) z (0, 0, 1) at (0.5, 0, 0)
named bodies: "tampa", "base"
